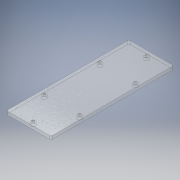
# Autodesk Inventor part: BT005_trajan20_21
Saved by Autodesk Inventor 2022.2 (Build 262287000, 287)
## iProperties
Company: HTBLA Kaindorf
RuleStatus: InUse
Created: 2022-08-07
Part Number: BT005_trajan20_21
Project: Zeichenmaschine_v2
Material: Acryl
Description: getriebemotor platte unten
Document SubType Name: Modeling
Designer: trajan20
Density: 1.188 g/cm^3
Appearance: Transparent - farblos
Mass: 123.67 g
Surface Area: 393.809 cm^2
Volume: 104.1 cm^3
AfterDocNew0: iProperties-Editor_aufrufen
Author: jan
Keywords: 2021
Autodesk Inventor part; units mm, degrees
ref_plane "YZ Plane" through (0, 0, 0) normal (1, 0, 0) x (0, 1, 0)
ref_plane "XZ Plane" through (0, 0, 0) normal (0, 1, 0) x (-1, 0, 0)
ref_plane "XY Plane" through (0, 0, 0) normal (0, 0, 1) x (1, 0, 0)
sketch "Skizze3" plane through (0, 0, 0) normal (0, 0, 1) x (1, 0, 0)
  line L0 (0, 0) -> (-220, 0)
  line L1 (-220, 0) -> (-220, 80)
  line L2 (-220, 80) -> (0, 80)
  line L3 (0, 80) -> (0, 0)
  line L4 (-60, 11.8952) -> (-60, -14.2347) construction
  line L5 (-11.7549, 40) -> (14.0889, 40) construction
  point P0 (-60, 8)
  point P1 (-8, 40)
  point P2 (0, 40)
  dimension "d4" = 80
  dimension "d5" = 220
  dimension "d27" = 60
  dimension "d28" = 8
  dimension "d29" = 8
  constraints: 12 end point, 3 point on line, 2 horizontal, 2 parallel, 1 midpoint, 1 perpendicular, 1 vertical
  measures "d4" distance between parallel lines of L0 L2
  measures "d5" distance between parallel lines of L1 L3
  measures "d27" distance between parallel lines of L3 L4
  measures "d28" distance from line of L3 point (-8, 40)
  measures "d29" distance from line of L0 point (-60, 8)
extrude "Extrusion3" add sketch "Skizze3" along normal blind 6
hole "Bohrung1" at (-60, 8, 0) at (-8, 40, 0) direction (0, 0, 1) diameter 4.5 end through all counterbore diameter 8 counterbore depth 4.4
ref_plane "Arbeitsebene1" through (-110, 80, 6) normal (-1, 0, 0) x (0, -1, 0)
ref_plane "Arbeitsebene2" through (-220, 40, 6) normal (0, -1, 0) x (1, 0, 0)
mirror "Spiegeln1" about plane through (-110, 80, 6) normal (-1, 0, 0) of "Bohrung1"
mirror "Spiegeln2" about plane through (-220, 40, 6) normal (0, -1, 0) of "Spiegeln1", "Bohrung1"
fillet "Rundung2" radius 2 4 edges at (0, 0, 3) (0, 80, 3) (-220, 80, 3) (-220, 0, 3)
